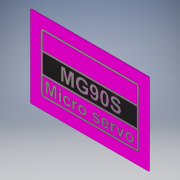
# Autodesk Inventor part: sticker
Saved by Autodesk Inventor 2019 (Build 230136000, 136)
## iProperties
Created: 2021-01-19
Part Number: sticker
Material: Generic
Document SubType Name: Modeling
Designer: CS
Density: 1 g/cm^3
Appearance: Magenta
Author: CS
Autodesk Inventor part; units mm, degrees
ref_plane "YZ Plane" through (0, 0, 0) normal (1, 0, 0) x (0, 1, 0)
ref_plane "XZ Plane" through (0, 0, 0) normal (0, 1, 0) x (-1, 0, 0)
ref_plane "XY Plane" through (0, 0, 0) normal (0, 0, 1) x (1, 0, 0)
sketch "Sketch1" plane through (0, 0, 0) normal (0, 0, 1) x (1, 0, 0)
  line L0 (7.25, -5) -> (-7.25, -5)
  line L1 (-7.25, -5) -> (-7.25, 5)
  line L2 (-7.25, 5) -> (7.25, 5)
  line L3 (7.25, 5) -> (7.25, -5)
  line L4 (7.25, -5) -> (-7.25, 5) construction
  line L5 (-7.25, -5) -> (7.25, 5) construction
  point P0 (0, 0)
  dimension "d0" = 14.5
  dimension "d1" = 10
  constraints: 12 end point, 2 midpoint, 2 parallel, 1 horizontal, 1 perpendicular
  measures "d0" distance of L1.end L2.end
  measures "d1" distance of L0.end L1.end
extrude "Extrusion1" add sketch "Sketch1" along normal blind 0.05
fillet "Fillet1" radius 0.1 4 edges at (7.25, 5, 0.025) (-7.25, 5, 0.025) (-7.25, -5, 0.025) (7.25, -5, 0.025)
sketch "Sketch3" plane through (0, 0, 0.05) normal (0, 0, 1) x (1, 0, 0)
  line L0 (5.65, -3.625) -> (-5.65, -3.625)
  line L1 (-6, -3.275) -> (-6, 3.275)
  line L2 (-5.65, 3.625) -> (5.65, 3.625)
  line L3 (6, 3.275) -> (6, -3.275)
  line L4 (6, -3.625) -> (-6, 3.625) construction
  line L5 (-6, -3.625) -> (6, 3.625) construction
  arc A0 (-5.65, 3.625) -> (-6, 3.275) centre (-5.65, 3.275) ccw
  arc A1 (6, 3.275) -> (5.65, 3.625) centre (5.65, 3.275) ccw
  arc A2 (5.65, -3.625) -> (6, -3.275) centre (5.65, -3.275) ccw
  arc A3 (-6, -3.275) -> (-5.65, -3.625) centre (-5.65, -3.275) ccw
  line L6 (5.65, 3.375) -> (-5.65, 3.375)
  arc A4 (-5.65, 3.375) -> (-5.75, 3.275) centre (-5.65, 3.275) ccw
  arc A5 (-5.75, -3.275) -> (-5.65, -3.375) centre (-5.65, -3.275) ccw
  line L7 (-5.65, -3.375) -> (5.65, -3.375)
  arc A6 (5.65, -3.375) -> (5.75, -3.275) centre (5.65, -3.275) ccw
  arc A7 (5.75, 3.275) -> (5.65, 3.375) centre (5.65, 3.275) ccw
  line L8 (5.75, -1.125) -> (-5.75, -1.125)
  line L9 (-5.75, -1.125) -> (-5.75, 1.125)
  line L10 (-5.75, 1.125) -> (5.75, 1.125)
  line L11 (5.75, 1.125) -> (5.75, -1.125)
  line L12 (5.75, -1.125) -> (-5.75, 1.125) construction
  line L13 (-5.75, -1.125) -> (5.75, 1.125) construction
  line L14 (-5.75, 1.125) -> (5.75, 1.125)
  line L15 (5.75, 1.375) -> (-5.75, 1.375)
  line L16 (5.75, -1.125) -> (-5.75, -1.125)
  line L17 (-5.75, -1.375) -> (5.75, -1.375)
  line L18 (-4.1649, 0.8418) -> (4.412, 0.8418) construction
  line L19 (4.412, 0.8418) -> (4.412, -1.0667) construction
  line L20 (4.412, -1.0667) -> (-4.1649, -1.0667) construction
  line L21 (-4.1649, -1.0667) -> (-4.1649, 0.8418) construction
  line L22 (-5.75, 3.275) -> (-5.75, 1.375)
  line L23 (-5.75, 1.125) -> (-5.75, -1.125)
  line L24 (-5.75, -1.375) -> (-5.75, -3.275)
  line L25 (5.75, 1.375) -> (5.75, 3.275)
  line L26 (5.75, -3.275) -> (5.75, -1.375)
  line L27 (5.75, -1.125) -> (5.75, 1.125)
  line L28 (-5.5366, -1.6727) -> (5.6464, -1.6727) construction
  line L29 (5.6464, -1.6727) -> (5.6464, -3.1686) construction
  line L30 (5.6464, -3.1686) -> (-5.5366, -3.1686) construction
  line L31 (-5.5366, -3.1686) -> (-5.5366, -1.6727) construction
  line L32 (-3.5057, -0.785) -> (-3.5057, 0.815)
  line L33 (-3.5057, 0.815) -> (-3.0215, 0.815)
  line L34 (-3.0215, 0.815) -> (-2.7325, -0.2765)
  line L35 (-2.7325, -0.2765) -> (-2.4484, 0.815)
  line L36 (-2.4484, 0.815) -> (-1.963, 0.815)
  line L37 (-1.963, 0.815) -> (-1.963, -0.785)
  line L38 (-1.963, -0.785) -> (-2.2618, -0.785)
  line L39 (-2.2618, -0.785) -> (-2.2618, 0.4748)
  line L40 (-2.2618, 0.4748) -> (-2.5789, -0.785)
  line L41 (-2.5789, -0.785) -> (-2.8911, -0.785)
  line L42 (-2.8911, -0.785) -> (-3.2057, 0.4748)
  line L43 (-3.2057, 0.4748) -> (-3.2069, -0.785)
  line L44 (-3.2069, -0.785) -> (-3.5057, -0.785)
  line L45 (-0.8959, -0.1984) -> (-0.8959, 0.0723)
  line L46 (-0.8959, 0.0723) -> (-0.1996, 0.0723)
  line L47 (-0.1996, 0.0723) -> (-0.1996, -0.5643)
  spline S0 degree 2 poles (-0.1996, -0.5643) (-0.3008, -0.663) (-0.6862, -0.8118) (-0.8837, -0.8118) knots 0 0 0 1 2 2 2
  spline S1 degree 2 poles (-0.8837, -0.8118) (-1.135, -0.8118) (-1.5081, -0.6009) (-1.6959, -0.2094) (-1.6959, 0.0199) knots 0 0 0 1 2 3 3 3
  spline S2 degree 2 poles (-1.6959, 0.0199) (-1.6959, 0.2699) (-1.4862, 0.6589) (-1.285, 0.7626) knots 0 0 0 1 2 2 2
  spline S3 degree 2 poles (-1.285, 0.7626) (-1.1301, 0.8418) (-0.9008, 0.8418) knots 0 0 0 1 1 1
  spline S4 degree 2 poles (-0.9008, 0.8418) (-0.6033, 0.8418) (-0.2679, 0.5918) (-0.2203, 0.3711) knots 0 0 0 1 2 2 2
  line L48 (-0.2203, 0.3711) -> (-0.5411, 0.3113)
  spline S5 degree 2 poles (-0.5411, 0.3113) (-0.5752, 0.4296) (-0.7618, 0.5662) (-0.9008, 0.5662) knots 0 0 0 1 2 2 2
  spline S6 degree 2 poles (-0.9008, 0.5662) (-1.113, 0.5662) (-1.363, 0.2979) (-1.363, 0.0333) knots 0 0 0 1 2 2 2
  spline S7 degree 2 poles (-1.363, 0.0333) (-1.363, -0.2509) (-1.1094, -0.5362) (-0.9045, -0.5362) knots 0 0 0 1 2 2 2
  spline S8 degree 2 poles (-0.9045, -0.5362) (-0.8033, -0.5362) (-0.5996, -0.4569) (-0.5264, -0.4009) knots 0 0 0 1 2 2 2
  line L49 (-0.5264, -0.4009) -> (-0.5264, -0.1984)
  line L50 (-0.5264, -0.1984) -> (-0.8959, -0.1984)
  line L51 (0.037, -0.413) -> (0.3333, -0.3801)
  spline S9 degree 2 poles (0.3333, -0.3801) (0.3443, -0.4704) (0.4358, -0.5582) (0.5114, -0.5582) knots 0 0 0 1 2 2 2
  spline S10 degree 2 poles (0.5114, -0.5582) (0.6065, -0.5582) (0.7394, -0.3838) (0.7577, -0.1082) knots 0 0 0 1 2 2 2
  spline S11 degree 2 poles (0.7577, -0.1082) (0.6431, -0.2423) (0.4687, -0.2423) knots 0 0 0 1 1 1
  spline S12 degree 2 poles (0.4687, -0.2423) (0.2809, -0.2423) (0.0065, 0.0479) (0.0065, 0.2809) knots 0 0 0 1 2 2 2
  spline S13 degree 2 poles (0.0065, 0.2809) (0.0065, 0.5235) (0.2955, 0.8211) (0.5199, 0.8211) knots 0 0 0 1 2 2 2
  spline S14 degree 2 poles (0.5199, 0.8211) (0.7626, 0.8211) (1.0748, 0.4443) (1.0748, 0.0138) knots 0 0 0 1 2 2 2
  spline S15 degree 2 poles (1.0748, 0.0138) (1.0748, -0.4252) (0.7492, -0.813) (0.4882, -0.813) knots 0 0 0 1 2 2 2
  spline S16 degree 2 poles (0.4882, -0.813) (0.3016, -0.813) (0.0699, -0.6118) (0.037, -0.413) knots 0 0 0 1 2 2 2
  spline S17 degree 2 poles (0.7309, 0.2552) (0.7309, 0.4028) (0.5943, 0.5662) (0.5053, 0.5662) knots 0 0 0 1 2 2 2
  spline S18 degree 2 poles (0.5053, 0.5662) (0.4199, 0.5662) (0.3077, 0.4321) (0.3077, 0.2809) knots 0 0 0 1 2 2 2
  spline S19 degree 2 poles (0.3077, 0.2809) (0.3077, 0.126) (0.4297, -0.0179) (0.5211, -0.0179) knots 0 0 0 1 2 2 2
  spline S20 degree 2 poles (0.5211, -0.0179) (0.6102, -0.0179) (0.7309, 0.1211) (0.7309, 0.2552) knots 0 0 0 1 2 2 2
  spline S21 degree 2 poles (1.7919, 0.8211) (2.0248, 0.8211) (2.1553, 0.6552) knots 0 0 0 1 1 1
  spline S22 degree 2 poles (2.1553, 0.6552) (2.3114, 0.4589) (2.3114, 0.004) knots 0 0 0 1 1 1
  spline S23 degree 2 poles (2.3114, 0.004) (2.3114, -0.4496) (2.1541, -0.6484) knots 0 0 0 1 1 1
  spline S24 degree 2 poles (2.1541, -0.6484) (2.0248, -0.8118) (1.7919, -0.8118) knots 0 0 0 1 1 1
  spline S25 degree 2 poles (1.7919, -0.8118) (1.5577, -0.8118) (1.2724, -0.4533) (1.2724, 0.0077) knots 0 0 0 1 2 2 2
  spline S26 degree 2 poles (1.2724, 0.0077) (1.2724, 0.4589) (1.4297, 0.6577) knots 0 0 0 1 1 1
  spline S27 degree 2 poles (1.4297, 0.6577) (1.5589, 0.8211) (1.7919, 0.8211) knots 0 0 0 1 1 1
  spline S28 degree 2 poles (1.7919, 0.5662) (1.7358, 0.5662) (1.6492, 0.4955) (1.6248, 0.404) knots 0 0 0 1 2 2 2
  spline S29 degree 2 poles (1.6248, 0.404) (1.5931, 0.2857) (1.5931, 0.004) knots 0 0 0 1 1 1
  spline S30 degree 2 poles (1.5931, 0.004) (1.5931, -0.2765) (1.6504, -0.4874) (1.7358, -0.5569) (1.7919, -0.5569) knots 0 0 0 1 2 3 3 3
  spline S31 degree 2 poles (1.7919, -0.5569) (1.848, -0.5569) (1.9345, -0.4862) (1.9589, -0.3948) knots 0 0 0 1 2 2 2
  spline S32 degree 2 poles (1.9589, -0.3948) (1.9906, -0.2765) (1.9906, 0.004) knots 0 0 0 1 1 1
  spline S33 degree 2 poles (1.9906, 0.004) (1.9906, 0.2857) (1.9333, 0.4955) (1.848, 0.5662) (1.7919, 0.5662) knots 0 0 0 1 2 3 3 3
  line L52 (2.5016, -0.263) -> (2.8163, -0.2326)
  spline S34 degree 2 poles (2.8163, -0.2326) (2.8443, -0.3911) (3.0187, -0.5399) (3.165, -0.5399) knots 0 0 0 1 2 2 2
  spline S35 degree 2 poles (3.165, -0.5399) (3.3211, -0.5399) (3.4797, -0.4082) (3.4797, -0.3191) knots 0 0 0 1 2 2 2
  spline S36 degree 2 poles (3.4797, -0.3191) (3.4797, -0.2618) (3.4126, -0.1826) (3.3297, -0.1533) knots 0 0 0 1 2 2 2
  spline S37 degree 2 poles (3.3297, -0.1533) (3.2736, -0.1338) (3.0711, -0.0838) knots 0 0 0 1 1 1
  spline S38 degree 2 poles (3.0711, -0.0838) (2.8114, -0.0191) (2.7065, 0.0748) knots 0 0 0 1 1 1
  spline S39 degree 2 poles (2.7065, 0.0748) (2.5589, 0.2065) (2.5589, 0.3955) knots 0 0 0 1 1 1
  spline S40 degree 2 poles (2.5589, 0.3955) (2.5589, 0.5187) (2.698, 0.7309) (2.9589, 0.8418) (3.1431, 0.8418) knots 0 0 0 1 2 3 3 3
  spline S41 degree 2 poles (3.1431, 0.8418) (3.4443, 0.8418) (3.7492, 0.5784) (3.7565, 0.3577) knots 0 0 0 1 2 2 2
  line L53 (3.7565, 0.3577) -> (3.4333, 0.3431)
  spline S42 degree 2 poles (3.4333, 0.3431) (3.4126, 0.4662) (3.276, 0.5748) (3.1394, 0.5748) knots 0 0 0 1 2 2 2
  spline S43 degree 2 poles (3.1394, 0.5748) (2.998, 0.5748) (2.9187, 0.5174) knots 0 0 0 1 1 1
  spline S44 degree 2 poles (2.9187, 0.5174) (2.8675, 0.4796) (2.8675, 0.4174) knots 0 0 0 1 1 1
  spline S45 degree 2 poles (2.8675, 0.4174) (2.8675, 0.3613) (2.915, 0.3199) knots 0 0 0 1 1 1
  spline S46 degree 2 poles (2.915, 0.3199) (2.9772, 0.2687) (3.4492, 0.1577) (3.6748, 0.0394) (3.8028, -0.1667) (3.8028, -0.3191) knots 0 0 0 1 2 3 4 4 4
  spline S47 degree 2 poles (3.8028, -0.3191) (3.8028, -0.4557) (3.6504, -0.696) (3.3711, -0.813) (3.1626, -0.813) knots 0 0 0 1 2 3 3 3
  spline S48 degree 2 poles (3.1626, -0.813) (2.8589, -0.813) (2.5333, -0.5326) (2.5016, -0.263) knots 0 0 0 1 2 2 2
  line L54 (-5.3969, -3.0727) -> (-5.3969, -1.6727)
  line L55 (-5.3969, -1.6727) -> (-4.9732, -1.6727)
  line L56 (-4.9732, -1.6727) -> (-4.7203, -2.6277)
  line L57 (-4.7203, -2.6277) -> (-4.4717, -1.6727)
  line L58 (-4.4717, -1.6727) -> (-4.047, -1.6727)
  line L59 (-4.047, -1.6727) -> (-4.047, -3.0727)
  line L60 (-4.047, -3.0727) -> (-4.3084, -3.0727)
  line L61 (-4.3084, -3.0727) -> (-4.3084, -1.9704)
  line L62 (-4.3084, -1.9704) -> (-4.5859, -3.0727)
  line L63 (-4.5859, -3.0727) -> (-4.859, -3.0727)
  line L64 (-4.859, -3.0727) -> (-5.1344, -1.9704)
  line L65 (-5.1344, -1.9704) -> (-5.1354, -3.0727)
  line L66 (-5.1354, -3.0727) -> (-5.3969, -3.0727)
  line L67 (-3.7664, -3.0727) -> (-3.7664, -2.0579)
  line L68 (-3.7664, -2.0579) -> (-3.4975, -2.0579)
  line L69 (-3.4975, -2.0579) -> (-3.4975, -3.0727)
  line L70 (-3.4975, -3.0727) -> (-3.7664, -3.0727)
  line L71 (-3.7664, -1.9213) -> (-3.7664, -1.6727)
  line L72 (-3.7664, -1.6727) -> (-3.4975, -1.6727)
  line L73 (-3.4975, -1.6727) -> (-3.4975, -1.9213)
  line L74 (-3.4975, -1.9213) -> (-3.7664, -1.9213)
  line L75 (-2.3408, -2.3578) -> (-2.6054, -2.4058)
  spline S49 degree 2 poles (-2.6054, -2.4058) (-2.6182, -2.3268) (-2.7132, -2.2468) (-2.7889, -2.2468) knots 0 0 0 1 2 2 2
  spline S50 degree 2 poles (-2.7889, -2.2468) (-2.8882, -2.2468) (-3.0077, -2.3855) (-3.0077, -2.5477) knots 0 0 0 1 2 2 2
  spline S51 degree 2 poles (-3.0077, -2.5477) (-3.0077, -2.728) (-2.886, -2.8764) (-2.7847, -2.8764) knots 0 0 0 1 2 2 2
  spline S52 degree 2 poles (-2.7847, -2.8764) (-2.7078, -2.8764) (-2.6107, -2.7889) (-2.5904, -2.6832) knots 0 0 0 1 2 2 2
  line L76 (-2.5904, -2.6832) -> (-2.3269, -2.728)
  spline S53 degree 2 poles (-2.3269, -2.728) (-2.3674, -2.9094) (-2.6011, -3.0951) (-2.7964, -3.0951) knots 0 0 0 1 2 2 2
  spline S54 degree 2 poles (-2.7964, -3.0951) (-3.0183, -3.0951) (-3.283, -2.8145) (-3.283, -2.5658) knots 0 0 0 1 2 2 2
  spline S55 degree 2 poles (-3.283, -2.5658) (-3.283, -2.3151) (-3.0183, -2.0355) (-2.7921, -2.0355) knots 0 0 0 1 2 2 2
  spline S56 degree 2 poles (-2.7921, -2.0355) (-2.6065, -2.0355) (-2.3888, -2.1945) (-2.3408, -2.3578) knots 0 0 0 1 2 2 2
  line L77 (-1.8787, -3.0727) -> (-2.1476, -3.0727)
  line L78 (-2.1476, -3.0727) -> (-2.1476, -2.0579)
  line L79 (-2.1476, -2.0579) -> (-1.8979, -2.0579)
  line L80 (-1.8979, -2.0579) -> (-1.8979, -2.202)
  spline S57 degree 2 poles (-1.8979, -2.202) (-1.8339, -2.0995) (-1.7325, -2.0355) (-1.6674, -2.0355) knots 0 0 0 1 2 2 2
  spline S58 degree 2 poles (-1.6674, -2.0355) (-1.5757, -2.0355) (-1.4914, -2.0867) knots 0 0 0 1 1 1
  line L81 (-1.4914, -2.0867) -> (-1.5735, -2.3204)
  spline S59 degree 2 poles (-1.5735, -2.3204) (-1.6418, -2.2767) (-1.6994, -2.2767) knots 0 0 0 1 1 1
  spline S60 degree 2 poles (-1.6994, -2.2767) (-1.756, -2.2767) (-1.8339, -2.3386) (-1.8787, -2.5008) (-1.8787, -2.7601) knots 0 0 0 1 2 3 3 3
  line L82 (-1.8787, -2.7601) -> (-1.8787, -3.0727)
  spline S61 degree 2 poles (-1.438, -2.5509) (-1.438, -2.4175) (-1.3057, -2.1668) (-1.0645, -2.0355) (-0.9151, -2.0355) knots 0 0 0 1 2 3 3 3
  spline S62 degree 2 poles (-0.9151, -2.0355) (-0.6847, -2.0355) (-0.3901, -2.3343) (-0.3901, -2.5626) knots 0 0 0 1 2 2 2
  spline S63 degree 2 poles (-0.3901, -2.5626) (-0.3901, -2.7921) (-0.6879, -3.0951) (-0.913, -3.0951) knots 0 0 0 1 2 2 2
  spline S64 degree 2 poles (-0.913, -3.0951) (-1.0528, -3.0951) (-1.3057, -2.9692) (-1.438, -2.7259) (-1.438, -2.5509) knots 0 0 0 1 2 3 3 3
  spline S65 degree 2 poles (-1.1627, -2.5648) (-1.1627, -2.7163) (-1.0197, -2.8764) (-0.9141, -2.8764) knots 0 0 0 1 2 2 2
  spline S66 degree 2 poles (-0.9141, -2.8764) (-0.8084, -2.8764) (-0.6665, -2.7163) (-0.6665, -2.5637) knots 0 0 0 1 2 2 2
  spline S67 degree 2 poles (-0.6665, -2.5637) (-0.6665, -2.4143) (-0.8084, -2.2543) (-0.9141, -2.2543) knots 0 0 0 1 2 2 2
  spline S68 degree 2 poles (-0.9141, -2.2543) (-1.0197, -2.2543) (-1.1627, -2.4143) (-1.1627, -2.5648) knots 0 0 0 1 2 2 2
  line L83 (0.2682, -2.7825) -> (0.5371, -2.7419)
  spline S69 degree 2 poles (0.5371, -2.7419) (0.5542, -2.8198) (0.6599, -2.9009) (0.7538, -2.9009) knots 0 0 0 1 2 2 2
  spline S70 degree 2 poles (0.7538, -2.9009) (0.8583, -2.9009) (0.9106, -2.8625) knots 0 0 0 1 1 1
  spline S71 degree 2 poles (0.9106, -2.8625) (0.9458, -2.8358) (0.9458, -2.791) knots 0 0 0 1 1 1
  spline S72 degree 2 poles (0.9458, -2.791) (0.9458, -2.7611) (0.9266, -2.7408) knots 0 0 0 1 1 1
  spline S73 degree 2 poles (0.9266, -2.7408) (0.9063, -2.7216) (0.837, -2.7056) knots 0 0 0 1 1 1
  spline S74 degree 2 poles (0.837, -2.7056) (0.5126, -2.6341) (0.4262, -2.5744) knots 0 0 0 1 1 1
  spline S75 degree 2 poles (0.4262, -2.5744) (0.3056, -2.4922) (0.3056, -2.3471) knots 0 0 0 1 1 1
  spline S76 degree 2 poles (0.3056, -2.3471) (0.3056, -2.2148) (0.5137, -2.0355) (0.7324, -2.0355) knots 0 0 0 1 2 2 2
  spline S77 degree 2 poles (0.7324, -2.0355) (0.9405, -2.0355) (1.1422, -2.171) (1.1806, -2.3044) knots 0 0 0 1 2 2 2
  line L84 (1.1806, -2.3044) -> (0.9277, -2.3514)
  spline S78 degree 2 poles (0.9277, -2.3514) (0.9117, -2.2916) (0.821, -2.2287) (0.7367, -2.2287) knots 0 0 0 1 2 2 2
  spline S79 degree 2 poles (0.7367, -2.2287) (0.631, -2.2287) (0.5862, -2.2585) knots 0 0 0 1 1 1
  spline S80 degree 2 poles (0.5862, -2.2585) (0.5553, -2.2788) (0.5553, -2.3129) knots 0 0 0 1 1 1
  spline S81 degree 2 poles (0.5553, -2.3129) (0.5553, -2.3407) (0.582, -2.361) knots 0 0 0 1 1 1
  spline S82 degree 2 poles (0.582, -2.361) (0.6182, -2.3876) (1.0461, -2.4847) (1.1304, -2.5562) knots 0 0 0 1 2 2 2
  spline S83 degree 2 poles (1.1304, -2.5562) (1.2147, -2.6277) (1.2147, -2.7558) knots 0 0 0 1 1 1
  spline S84 degree 2 poles (1.2147, -2.7558) (1.2147, -2.8945) (0.9821, -3.0951) (0.7538, -3.0951) knots 0 0 0 1 2 2 2
  spline S85 degree 2 poles (0.7538, -3.0951) (0.5467, -3.0951) (0.3056, -2.9265) (0.2682, -2.7825) knots 0 0 0 1 2 2 2
  line L85 (2.0374, -2.7494) -> (2.3053, -2.7942)
  spline S86 degree 2 poles (2.3053, -2.7942) (2.2541, -2.9415) (2.031, -3.0951) (1.8635, -3.0951) knots 0 0 0 1 2 2 2
  spline S87 degree 2 poles (1.8635, -3.0951) (1.5989, -3.0951) (1.4719, -2.9222) knots 0 0 0 1 1 1
  spline S88 degree 2 poles (1.4719, -2.9222) (1.3716, -2.7835) (1.3716, -2.5733) knots 0 0 0 1 1 1
  spline S89 degree 2 poles (1.3716, -2.5733) (1.3716, -2.3204) (1.6352, -2.0355) (1.8368, -2.0355) knots 0 0 0 1 2 2 2
  spline S90 degree 2 poles (1.8368, -2.0355) (2.0631, -2.0355) (2.3245, -2.3343) (2.3192, -2.6427) knots 0 0 0 1 2 2 2
  line L86 (2.3192, -2.6427) -> (1.6469, -2.6427)
  spline S91 degree 2 poles (1.6469, -2.6427) (1.6501, -2.7622) (1.7739, -2.8945) (1.8667, -2.8945) knots 0 0 0 1 2 2 2
  spline S92 degree 2 poles (1.8667, -2.8945) (1.9297, -2.8945) (2.015, -2.8262) (2.0374, -2.7494) knots 0 0 0 1 2 2 2
  spline S93 degree 2 poles (2.0524, -2.4783) (2.0492, -2.362) (1.935, -2.2404) (1.8528, -2.2404) knots 0 0 0 1 2 2 2
  spline S94 degree 2 poles (1.8528, -2.2404) (1.7653, -2.2404) (1.7077, -2.3044) knots 0 0 0 1 1 1
  spline S95 degree 2 poles (1.7077, -2.3044) (1.6512, -2.3684) (1.6512, -2.4783) knots 0 0 0 1 1 1
  line L87 (1.6512, -2.4783) -> (2.0524, -2.4783)
  line L88 (2.7951, -3.0727) -> (2.5262, -3.0727)
  line L89 (2.5262, -3.0727) -> (2.5262, -2.0579)
  line L90 (2.5262, -2.0579) -> (2.7759, -2.0579)
  line L91 (2.7759, -2.0579) -> (2.7759, -2.202)
  spline S96 degree 2 poles (2.7759, -2.202) (2.8399, -2.0995) (2.9413, -2.0355) (3.0063, -2.0355) knots 0 0 0 1 2 2 2
  spline S97 degree 2 poles (3.0063, -2.0355) (3.0981, -2.0355) (3.1824, -2.0867) knots 0 0 0 1 1 1
  line L92 (3.1824, -2.0867) -> (3.1003, -2.3204)
  spline S98 degree 2 poles (3.1003, -2.3204) (3.032, -2.2767) (2.9743, -2.2767) knots 0 0 0 1 1 1
  spline S99 degree 2 poles (2.9743, -2.2767) (2.9178, -2.2767) (2.8399, -2.3386) (2.7951, -2.5008) (2.7951, -2.7601) knots 0 0 0 1 2 3 3 3
  line L93 (2.7951, -2.7601) -> (2.7951, -3.0727)
  line L94 (3.5772, -3.0727) -> (3.1696, -2.0579)
  line L95 (3.1696, -2.0579) -> (3.4513, -2.0579)
  line L96 (3.4513, -2.0579) -> (3.6423, -2.5754)
  line L97 (3.6423, -2.5754) -> (3.6978, -2.7483)
  spline S100 degree 2 poles (3.6978, -2.7483) (3.7192, -2.6832) (3.7245, -2.6619) knots 0 0 0 1 1 1
  spline S101 degree 2 poles (3.7245, -2.6619) (3.7384, -2.6192) (3.7533, -2.5754) knots 0 0 0 1 1 1
  line L98 (3.7533, -2.5754) -> (3.9464, -2.0579)
  line L99 (3.9464, -2.0579) -> (4.2228, -2.0579)
  line L100 (4.2228, -2.0579) -> (3.8195, -3.0727)
  line L101 (3.8195, -3.0727) -> (3.5772, -3.0727)
  spline S102 degree 2 poles (4.3231, -2.5509) (4.3231, -2.4175) (4.4554, -2.1668) (4.6966, -2.0355) (4.846, -2.0355) knots 0 0 0 1 2 3 3 3
  spline S103 degree 2 poles (4.846, -2.0355) (5.0765, -2.0355) (5.371, -2.3343) (5.371, -2.5626) knots 0 0 0 1 2 2 2
  spline S104 degree 2 poles (5.371, -2.5626) (5.371, -2.7921) (5.0733, -3.0951) (4.8481, -3.0951) knots 0 0 0 1 2 2 2
  spline S105 degree 2 poles (4.8481, -3.0951) (4.7083, -3.0951) (4.4554, -2.9692) (4.3231, -2.7259) (4.3231, -2.5509) knots 0 0 0 1 2 3 3 3
  spline S106 degree 2 poles (4.5984, -2.5648) (4.5984, -2.7163) (4.7414, -2.8764) (4.8471, -2.8764) knots 0 0 0 1 2 2 2
  spline S107 degree 2 poles (4.8471, -2.8764) (4.9527, -2.8764) (5.0946, -2.7163) (5.0946, -2.5637) knots 0 0 0 1 2 2 2
  spline S108 degree 2 poles (5.0946, -2.5637) (5.0946, -2.4143) (4.9527, -2.2543) (4.8471, -2.2543) knots 0 0 0 1 2 2 2
  spline S109 degree 2 poles (4.8471, -2.2543) (4.7414, -2.2543) (4.5984, -2.4143) (4.5984, -2.5648) knots 0 0 0 1 2 2 2
  point P0 (0, 0)
  dimension "d51" = 12
  dimension "d52" = 7.25
  dimension "d53" = 0.35
  dimension "d54" = 0.25
  dimension "d55" = 0.25
  dimension "d56" = 0.25
  dimension "d57" = 2.25
  dimension "d64" = 0.25
  dimension "d65" = 0.25
  constraints: 48 end point, 16 parallel, 16 point on circle, 8 centre point, 8 point on line, 8 tangent, 5 perpendicular, 4 collinear, 4 equal radius, 4 horizontal, 4 midpoint, 7 other
  measures "d51" distance of L4.end L5.end
  measures "d52" distance of L5.end L4.start
  measures "d53" radius of A0
  measures "d54" distance between parallel lines of L2 L6
  measures "d55" distance between parallel lines of L15 L14
  measures "d56" distance between parallel lines of L16 L17
  measures "d57" distance between parallel lines of L14 L8
  measures "d64" distance between parallel lines of L1 L22
  measures "d65" distance between parallel lines of L0 L7
extrude "Extrusion3" cut sketch "Sketch3" against normal blind 0.0001
equation "\"d55\" = d54"
equation "\"d56\" = d55"
equation "\"d65\" = d64"
body "Solid1"
